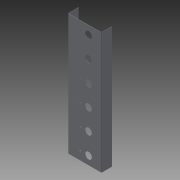
# Autodesk Inventor part: obudowa nowa
Saved by Autodesk Inventor 2015 (Build 190159000, 159)
## iProperties
Created: 2015-11-08
Part Number: obudowa nowa
Material: Generic
Document SubType Name: Sheet Metal
Designer: Komp
Density: 1 g/cm^3
Flat Pattern Width: 12.8262 cm
Flat Pattern Length: 29 cm
Flat Pattern Area: 371.96 cm^2
Sheet Metal Rule: Default_mm
Sheet Metal Width: 128,262 mm
Sheet Metal Length: 290,000 mm
Sheet Metal Area: 37195,965 mm^2
Appearance: Default
Author: Komp
Autodesk Inventor part; units mm, degrees
ref_plane "YZ Plane" through (0, 0, 0) normal (1, 0, 0) x (0, 1, 0)
ref_plane "XZ Plane" through (0, 0, 0) normal (0, 1, 0) x (-1, 0, 0)
ref_plane "XY Plane" through (0, 0, 0) normal (0, 0, 1) x (1, 0, 0)
sketch "Sketch1" plane through (0, 0, 0) normal (0, 1, 0) x (-1, 0, 0)
  line L0 (40, 131.7658) -> (-40, 131.7658)
  line L1 (-40, 131.7658) -> (-40, -158.2342)
  line L2 (-40, -158.2342) -> (40, -158.2342)
  line L3 (40, -158.2342) -> (40, 131.7658)
  point P0 (0, 0)
  dimension "d0" = 80
  dimension "d1" = 290
  measures "d0" distance of L0.start L0.end
  measures "d1" distance of L2.end L0.start
extrude "Plate1" add sketch "Sketch1" along normal blind 0.5
sketch "Sketch2" plane through (39.5, 0, -158.2342) normal (1, 0, 0) x (0, 1, 0)
  line L0 (0, 290) -> (0, 0)
  line L1 (0, 0) -> (25, 0)
  line L2 (25, 0) -> (25, 290)
  line L3 (25, 290) -> (0, 290)
  constraints: 6 end point, 1 horizontal, 1 perpendicular, 1 vertical
edge flange "Flange1" height 25 angle 90 thickness 0.5 bend radius 0.5 thickness toward (1, 0, 0) relief tear relief width 0.5 relief depth 0.25 edges at (40, 0.5, -13.2342) wall of the first edge with corners at (39.5, 0, 131.7658) (39.5, 0, -158.2342) (39.5, 25, -158.2342) (39.5, 25, 131.7658)
bend "Bend1"
corner "Corner1"
sketch "Sketch3" plane through (-39.5, 0, 131.7658) normal (-1, 0, 0) x (0, -1, 0)
  line L0 (0, -290) -> (0, 0)
  line L1 (0, 0) -> (-25, 0)
  line L2 (-25, 0) -> (-25, -290)
  line L3 (-25, -290) -> (0, -290)
  constraints: 6 end point, 1 horizontal, 1 perpendicular, 1 vertical
edge flange "Flange2" height 25 angle 90 thickness 0.5 bend radius 0.5 thickness toward (-1, 0, 0) relief tear relief width 0.5 relief depth 0.25 edges at (-40, 0.5, -13.2342) wall of the first edge with corners at (-39.5, 0, -158.2342) (-39.5, 0, 131.7658) (-39.5, 25, 131.7658) (-39.5, 25, -158.2342)
bend "Bend2"
corner "Corner2"
hole "Hole1" at (9, 0, -138.2342) direction (0, 1, 0) diameter 16 depth 0.5 tip angle 118
hole "Hole2" at (9, 0, -88.2342) direction (0, 1, 0) diameter 16 depth 0.5 tip angle 118
hole "Hole3" at (9, 0, -38.2342) direction (0, 1, 0) diameter 16 depth 0.5 tip angle 118
hole "Hole4" at (9, 0, 11.7658) direction (0, 1, 0) diameter 16 depth 0.5 tip angle 118
hole "Hole5" at (9, 0, 61.7658) direction (0, 1, 0) diameter 16 depth 0.5 tip angle 118
hole "Hole6" at (9, 0, 111.7658) direction (0, 1, 0) diameter 16 depth 0.5 tip angle 118
hole "Hole7" at (-11, 0, -138.2342) direction (0, 1, 0) diameter 3 depth 0.5 tip angle 118
hole "Hole8" at (-11, 0, -88.2342) direction (0, 1, 0) diameter 3 depth 0.5 tip angle 118
hole "Hole9" at (-11, 0, -38.2342) direction (0, 1, 0) diameter 3 depth 0.5 tip angle 118
hole "Hole10" at (-11, 0, 11.7658) direction (0, 1, 0) diameter 3 depth 0.5 tip angle 118
hole "Hole11" at (-11, 0, 61.7658) direction (0, 1, 0) diameter 3 depth 0.5 tip angle 118
hole "Hole12" at (-11, 0, 111.7658) direction (0, 1, 0) diameter 3 depth 0.5 tip angle 118
hole "Hole13" at (-29, 0, -13.2342) direction (0, 1, 0) diameter 3 depth 0.5 tip angle 118
hole "Hole14" at (-29, 0, -23.2342) direction (0, 1, 0) diameter 3 depth 0.5 tip angle 118
hole "Hole15" at (-29, 0, -3.2342) direction (0, 1, 0) diameter 3 depth 0.5 tip angle 118
hole "Hole16" at (-40, 13, 91.7658) direction (1, 0, 0) diameter 10 depth 0.5 tip angle 118
hole "Hole17" at (-40, 13, 76.7658) direction (1, 0, 0) diameter 2 depth 0.5 tip angle 118
hole "Hole18" at (-40, 13, 53.7658) direction (1, 0, 0) diameter 2 depth 0.5 tip angle 118
sketch "Sketch4" plane through (-40, 25, -158.2342) normal (-1, 0, 0) x (0, 0, 1)
  line L0 (229, -15) -> (217, -15)
  line L1 (217, -15) -> (217, -9)
  line L2 (217, -9) -> (229, -9)
  line L3 (229, -9) -> (229, -15)
  line L4 (290, 0) -> (290, -24) projected
  point P0 (158.2342, -25)
  dimension "d185" = 61
  dimension "d186" = 73
  constraints: 8 end point, 2 parallel, 1 horizontal, 1 perpendicular
  measures "d185" distance between parallel lines of L4 L3
  measures "d186" distance between parallel lines of L4 L1
extrude "Cut1" cut sketch "Sketch4" against normal blind 0.5
sketch "Sketch5" plane through (-40, 25, -158.2342) normal (-1, 0, 0) x (0, 0, 1)
  line L0 (198.5735, -16.892) -> (191.5735, -16.892)
  line L1 (191.5735, -16.892) -> (191.5735, -19.892)
  line L2 (191.5735, -19.892) -> (198.5735, -19.892)
  line L3 (198.5735, -19.892) -> (198.5735, -16.892)
  point P0 (158.2342, -25)
  dimension "d189" = 3
  dimension "d190" = 7
  constraints: 8 end point, 2 parallel, 1 perpendicular
  measures "d189" distance between parallel lines of L0 L2
  measures "d190" distance between parallel lines of L1 L3
extrude "Cut2" cut sketch "Sketch5" against normal blind 0.5
hole "Hole19" at (-40, 13, 11.7658) direction (1, 0, 0) diameter 16 depth 0.5 tip angle 118
hole "Hole20" at (-40, 13, 23.0658) direction (1, 0, 0) diameter 3 depth 0.5 tip angle 118
hole "Hole21" at (-40, 13, 0.4658) direction (1, 0, 0) diameter 3 depth 0.5 tip angle 118
equation "\"d30\" = Thickness"
equation "\"d39\" = Thickness"
equation "\"d48\" = Thickness"
equation "\"d57\" = Thickness"
equation "\"d66\" = Thickness"
equation "\"d75\" = Thickness"
equation "\"d84\" = Thickness"
equation "\"d93\" = Thickness"
equation "\"d102\" = Thickness"
equation "\"d111\" = Thickness"
equation "\"d120\" = Thickness"
equation "\"d129\" = Thickness"
equation "\"d138\" = Thickness"
equation "\"d147\" = Thickness"
equation "\"d156\" = Thickness"
equation "\"d165\" = Thickness"
equation "\"d174\" = Thickness"
equation "\"d183\" = Thickness"
equation "\"d187\" = Thickness"
equation "\"d191\" = Thickness"
equation "\"d200\" = Thickness"
equation "\"d209\" = Thickness"
equation "\"d219\" = Thickness"
equation "\"d3\" = BendReliefWidth"
equation "\"d4\" = BendReliefDepth"
equation "\"d5\" = MinimumRemnant"
equation "\"d6\" = BendRadius"
equation "\"d9\" = BendRadius"
equation "\"d10\" = CornerReliefSize"
equation "\"d11\" = GapSize"
equation "\"d12\" = JacobiRadiusSize"
equation "\"d13\" = BendReliefWidth"
equation "\"d14\" = BendReliefDepth"
equation "\"d15\" = MinimumRemnant"
equation "\"d16\" = BendRadius"
equation "\"d19\" = BendRadius"
equation "\"d20\" = CornerReliefSize"
equation "\"d21\" = GapSize"
equation "\"d22\" = JacobiRadiusSize"
equation "\"BendRadius\" = Thickness"
equation "\"BendReliefWidth\" = Thickness"
equation "\"BendReliefDepth\" = 0.5 * Thickness"
equation "\"CornerReliefSize\" = 4 * Thickness"
equation "\"MinimumRemnant\" = 2 * Thickness"
equation "\"TransitionRadius\" = BendRadius"
equation "\"JacobiRadiusSize\" = BendRadius"
equation "\"GapSize\" = Thickness"
equation "\"d2\" = BendRadius"
equation "\"Thickness\" = 0.5"
body "Solid1"
